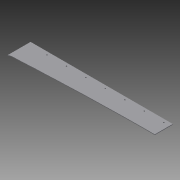
# Autodesk Inventor part: profil masca dreapta
Saved by Autodesk Inventor 2015 SP1 (Build 190203100, 203)
## iProperties
Created: 2015-10-20
Part Number: profil masca dreapta
Material: Generic
Document SubType Name: Modeling
Designer: ubik
Density: 1 g/cm^3
Appearance: Default
Author: ubik
Autodesk Inventor part; units mm, degrees
ref_plane "YZ Plane" through (0, 0, 0) normal (1, 0, 0) x (0, 1, 0)
ref_plane "XZ Plane" through (0, 0, 0) normal (0, 1, 0) x (-1, 0, 0)
ref_plane "XY Plane" through (0, 0, 0) normal (0, 0, 1) x (1, 0, 0)
sketch "Sketch1" plane through (0, 0, 0) normal (0, 0, 1) x (1, 0, 0)
  line L0 (5.4169, -0.155) -> (5.4169, 3.485) construction
  line L1 (20, 0) -> (20, 4.5) construction
  line L2 (30, 0) -> (30, 4.85) construction
  line L3 (40, 0) -> (40, 5.35) construction
  line L4 (50, 0) -> (50, 5.89) construction
  line L5 (60, 0) -> (60, 6.34) construction
  line L6 (70, 0) -> (70, 6.97) construction
  line L7 (80, 0) -> (80, 7.27) construction
  line L8 (89.0098, -0.188) -> (89.0098, 7.492) construction
  line L9 (100, 0) -> (100, 8.03) construction
  line L10 (110, 0) -> (110, 8.48) construction
  line L11 (120, 0) -> (120, 9) construction
  line L12 (130, 0) -> (130, 9.28) construction
  line L13 (140, 0) -> (140, 9.6) construction
  line L14 (150, 0) -> (150, 10.14) construction
  line L15 (160, 0) -> (160, 10.3) construction
  line L16 (170, 0) -> (170, 10.9) construction
  line L17 (180, 0) -> (180, 11.14) construction
  line L18 (190, 0) -> (190, 11.48) construction
  line L19 (200, 0) -> (200, 11.72) construction
  line L20 (210, 0) -> (210, 11.91) construction
  line L21 (220, 0) -> (220, 12.02) construction
  line L22 (230, 0) -> (230, 12.41) construction
  line L23 (240, 0) -> (240, 12.58) construction
  line L24 (250, 0) -> (250, 12.8) construction
  line L25 (260, 0) -> (260, 13.2) construction
  line L26 (270, 0) -> (270, 13.17) construction
  line L27 (280, 0) -> (280, 13.34) construction
  line L28 (290, 0) -> (290, 13.48) construction
  line L29 (300, 0) -> (300, 13.62) construction
  line L30 (310, 0) -> (310, 13.72) construction
  line L31 (320, 0) -> (320, 13.78) construction
  line L32 (329.0907, 0) -> (329.0907, 13.84) construction
  line L33 (340, 0) -> (340, 13.94) construction
  line L34 (350, 0) -> (350, 13.84) construction
  line L35 (360, 0) -> (360, 13.78) construction
  line L36 (369.2114, -0.0184) -> (369.2114, 13.6816) construction
  line L37 (380, 0) -> (380, 13.65) construction
  line L38 (390, 0) -> (390, 13.6) construction
  line L39 (400, 0) -> (401, 0) construction
  line L40 (400, 0) -> (400, 13.55) construction
  line L41 (410, 0) -> (410, 13.5) construction
  line L42 (420, 0) -> (420, 13.45) construction
  line L43 (430, 0) -> (430, 13.4) construction
  line L44 (440, 0) -> (440, 13.3) construction
  line L45 (449.0907, 0.4814) -> (449.0907, 13.6014) construction
  line L46 (459.0907, 0.4814) -> (459.0907, 13.3914) construction
  line L47 (469.0907, 0.4814) -> (469.0907, 13.2414) construction
  line L48 (480, 0) -> (480, 12.68) construction
  line L49 (490, 0) -> (490, 12.44) construction
  line L50 (500, 0) -> (500, 12.3) construction
  line L51 (509.0907, -0.2033) -> (509.0907, 12.0967) construction
  line L52 (520, 0) -> (520, 11.72) construction
  line L53 (530, 0) -> (530, 11.57) construction
  line L54 (540, 0) -> (540, 11.42) construction
  line L55 (550, 0) -> (550, 11.11) construction
  line L56 (560, 0) -> (560, 10.82) construction
  line L57 (570, 0) -> (570, 10.59) construction
  line L58 (580, 0) -> (580, 10.1) construction
  line L59 (590, 0) -> (590, 9.83) construction
  line L60 (600, 0) -> (600, 9.58) construction
  line L61 (610, 0) -> (610, 8.82) construction
  line L62 (620, 0) -> (620, 8.44) construction
  line L63 (630, 0) -> (630, 8.19) construction
  line L64 (640, 0) -> (640, 7.4) construction
  line L65 (650, 0) -> (650, 7.17) construction
  line L66 (660, 0) -> (660, 6.6) construction
  line L67 (670, 0) -> (670, 5.98) construction
  line L68 (680, 0) -> (680, 5.6) construction
  line L69 (690, 0) -> (690, 4.88) construction
  line L70 (700, 0) -> (700, 4.66) construction
  line L71 (710, 0) -> (710, 4.2) construction
  line L72 (723.6522, 0) -> (723.6522, 3.65) construction
  spline S0 degree 4 poles (365, 13.7179) (367.2861, 13.6927) (372.0134, 13.6545) (380.3551, 13.6692) (389.8057, 13.5915) (400.0956, 13.558) (410.0033, 13.4823) (421.3768, 13.4934) (429.3322, 13.2433) (449.7646, 13.8639) (457.9068, 13.2204) (468.9537, 13.4987) (480.036, 12.5023) (489.6496, 12.4681) (500.2854, 12.2919) (508.8725, 12.1726) (520.2953, 11.6164) (529.8107, 11.5877) (540.0222, 11.4708) (549.9829, 11.1082) (560.0057, 10.7542) (570.0019, 10.7332) (579.9984, 9.9959) (589.9997, 9.777) (600.0116, 9.8283) (609.9915, 8.641) (619.9979, 8.3459) (630.0125, 8.5241) (639.9877, 7.0259) (650.0051, 7.4074) (660.0056, 6.5957) (669.9819, 5.8092) (680.0431, 5.8817) (689.9966, 4.5194) (704.3323, 5.0971) (713.673, 3.1501) (728.99, 5.1632) (730, 0) knots 0 0 0 0 0 0.02684 0.054659 0.082757 0.110587 0.138416 0.168902 0.199388 0.229874 0.260674 0.28882 0.316965 0.344787 0.372606 0.400425 0.428244 0.456387 0.48422 0.512054 0.539892 0.567729 0.595565 0.623411 0.651255 0.679099 0.706953 0.734798 0.762646 0.790499 0.818344 0.846197 0.874046 0.901891 0.930909 1 1 1 1 1
  line L73 (730, 0) -> (730, -8)
  line L74 (0, -8) -> (0, 0)
  line L75 (730, 0) -> (730, 30)
  line L76 (0, 30) -> (0, 0)
  line L77 (365, 30) -> (365, 13.7179)
  spline S1 degree 4 poles (0, 0) (0.0145, 4.4252) (16.695, 4.2728) (25.5931, 4.6367) (39.9968, 5.308) (49.9359, 5.9756) (60.0423, 6.2013) (69.7712, 7.1165) (80.3142, 7.2834) (88.7823, 7.3775) (100.3206, 8.1188) (109.7967, 8.3884) (120.0179, 9.1072) (129.981, 9.2863) (140.0119, 9.4298) (149.9908, 10.4309) (160.0093, 9.9672) (169.9914, 11.1789) (180.002, 10.9851) (189.9972, 11.578) (200.0002, 11.675) (209.999, 12.0061) (220.0034, 11.8503) (229.9974, 12.5451) (240.0006, 12.5626) (250.002, 12.6657) (259.9971, 13.4447) (269.9981, 12.9993) (280.0064, 13.4149) (289.9803, 13.4487) (300.0251, 13.6425) (309.7904, 13.7216) (320.3191, 13.7927) (328.7925, 13.7961) (340.3354, 14.0383) (349.4183, 13.7716) (359.7782, 13.8198) (362.7638, 13.7425) (365, 13.7179) knots 0 0 0 0 0 0.066978 0.095643 0.122888 0.150138 0.177385 0.204282 0.231509 0.258733 0.28596 0.313533 0.340775 0.368018 0.395257 0.4225 0.449743 0.476983 0.504224 0.531459 0.558693 0.585928 0.613162 0.640396 0.667633 0.694868 0.722102 0.749336 0.776568 0.8038 0.831031 0.857945 0.885162 0.912379 0.939595 0.965135 1 1 1 1 1
  line L78 (291.4223, 14.5287) -> (438.5777, 12.907) construction
  arc A0 (306.255, 16.0656) -> (423.7824, 14.7704) centre (376.201, 1030.1036) ccw construction
  line L79 (291.4223, 14.5287) -> (438.5777, 12.907) construction
  arc A1 (307.6611, 20.7672) -> (422.4803, 19.5019) centre (367.8656, 273.7464) ccw construction
  line L80 (365, 13.7179) -> (365, 0)
  line L81 (365, 0) -> (365, 60)
  line L82 (365, 60) -> (0, 60)
  line L83 (0, 60) -> (0, 0)
  dimension "d0" = 730
  dimension "d1" = 3.64
  dimension "d2" = 4.5
  dimension "d3" = 4.85
  dimension "d4" = 5.35
  dimension "d5" = 5.89
  dimension "d6" = 6.34
  dimension "d7" = 6.97
  dimension "d8" = 7.27
  dimension "d9" = 7.68
  dimension "d10" = 8.03
  dimension "d11" = 8.48
  dimension "d12" = 9
  dimension "d13" = 9.28
  dimension "d14" = 9.6
  dimension "d15" = 10.14
  dimension "d16" = 10.3
  dimension "d17" = 10.9
  dimension "d18" = 11.14
  dimension "d19" = 11.48
  dimension "d20" = 11.72
  dimension "d21" = 11.91
  dimension "d22" = 12.02
  dimension "d23" = 12.41
  dimension "d24" = 12.58
  dimension "d25" = 12.8
  dimension "d26" = 13.2
  dimension "d27" = 13.17
  dimension "d28" = 13.34
  dimension "d29" = 13.48
  dimension "d30" = 13.62
  dimension "d31" = 13.72
  dimension "d32" = 13.78
  dimension "d34" = 13.84
  dimension "d35" = 13.94
  dimension "d36" = 13.84
  dimension "d37" = 13.78
  dimension "d38" = 13.7
  dimension "d39" = 13.65
  dimension "d40" = 13.6
  dimension "d41" = 13.55
  dimension "d42" = 13.5
  dimension "d43" = 13.45
  dimension "d44" = 13.4
  dimension "d45" = 13.3
  dimension "d47" = 13.12
  dimension "d48" = 12.91
  dimension "d49" = 12.76
  dimension "d50" = 12.68
  dimension "d51" = 12.44
  dimension "d52" = 12.3
  dimension "d53" = 12.3
  dimension "d54" = 11.72
  dimension "d55" = 11.57
  dimension "d56" = 11.42
  dimension "d57" = 11.11
  dimension "d58" = 10.82
  dimension "d59" = 10.59
  dimension "d60" = 10.1
  dimension "d61" = 9.83
  dimension "d62" = 9.58
  dimension "d63" = 8.82
  dimension "d64" = 8.44
  dimension "d65" = 8.19
  constraints: 168 end point, 63 vertical, 6 midpoint, 6 parallel, 2 centre point, 2 point on circle, 80 other
  measures "d0" distance of L74.end point (730, 0)
  measures "d1" distance of L0.start L0.end
  measures "d2" distance of L1.start L1.end
  measures "d3" distance of L2.start L2.end
  measures "d4" distance of L3.start L3.end
  measures "d5" distance of L4.start L4.end
  measures "d6" distance of L5.start L5.end
  measures "d7" distance of L6.start L6.end
  measures "d8" distance of L7.start L7.end
  measures "d9" distance of L8.start L8.end
  measures "d10" distance of L9.start L9.end
  measures "d11" distance of L10.start L10.end
  measures "d12" distance of L11.start L11.end
  measures "d13" distance of L12.start L12.end
  measures "d14" distance of L13.start L13.end
  measures "d15" distance of L14.start L14.end
  measures "d16" distance of L15.start L15.end
  measures "d17" distance of L16.start L16.end
  measures "d18" distance of L17.start L17.end
  measures "d19" distance of L18.start L18.end
  measures "d20" distance of L19.start L19.end
  measures "d21" distance of L20.start L20.end
  measures "d22" distance of L21.start L21.end
  measures "d23" distance of L22.start L22.end
  measures "d24" distance of L23.start L23.end
  measures "d25" distance of L24.start L24.end
  measures "d26" distance of L25.start L25.end
  measures "d27" distance of L26.start L26.end
  measures "d28" distance of L27.start L27.end
  measures "d29" distance of L28.start L28.end
  measures "d30" distance of L29.start L29.end
  measures "d31" distance of L30.start L30.end
  measures "d32" distance of L31.start L31.end
  measures "d34" distance of L32.start L32.end
  measures "d35" distance of L33.start L33.end
  measures "d36" distance of L34.start L34.end
  measures "d37" distance of L35.start L35.end
  measures "d38" distance of L36.start L36.end
  measures "d39" distance of L37.start L37.end
  measures "d40" distance of L38.start L38.end
  measures "d41" distance of L39.start L40.end
  measures "d42" distance of L41.start L41.end
  measures "d43" distance of L42.start L42.end
  measures "d44" distance of L43.start L43.end
  measures "d45" distance of L44.start L44.end
  measures "d47" distance of L45.start L45.end
  measures "d48" distance of L46.start L46.end
  measures "d49" distance of L47.start L47.end
  measures "d50" distance of L48.start L48.end
  measures "d51" distance of L49.start L49.end
  measures "d52" distance of L50.start L50.end
  measures "d53" distance of L51.start L51.end
  measures "d54" distance of L52.start L52.end
  measures "d55" distance of L53.start L53.end
  measures "d56" distance of L54.start L54.end
  measures "d57" distance of L55.start L55.end
  measures "d58" distance of L56.start L56.end
  measures "d59" distance of L57.start L57.end
  measures "d60" distance of L58.start L58.end
  measures "d61" distance of L59.start L59.end
  measures "d62" distance of L60.start L60.end
  measures "d63" distance of L61.start L61.end
  measures "d64" distance of L62.start L62.end
  measures "d65" distance of L63.start L63.end
extrude "Extrusion2" add sketch "Sketch1" along normal blind 1.5
hole "Hole1" at (50, 52, 1.5) direction (0, 0, -1) diameter 3 end through all
hole "Hole2" at (100, 52, 1.5) direction (0, 0, -1) diameter 3 end through all
hole "Hole3" at (150, 52, 1.5) direction (0, 0, -1) diameter 3 end through all
hole "Hole4" at (200, 52, 1.5) direction (0, 0, -1) diameter 3 end through all
hole "Hole5" at (250, 52, 1.5) direction (0, 0, -1) diameter 3 end through all
hole "Hole6" at (300, 52, 1.5) direction (0, 0, -1) diameter 3 end through all
hole "Hole7" at (350, 52, 1.5) direction (0, 0, -1) diameter 3 end through all
body "Solid2"
